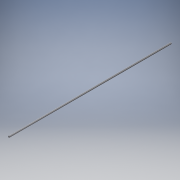
# Autodesk Inventor part: PIVOT WIRE
Saved by Autodesk Inventor 2016 (Build 200138000, 138)
## iProperties
Created: 2015-09-17
Part Number: PIVOT WIRE
Material: Steel, Mild
Document SubType Name: Modeling
Designer: testing
Density: 7.86 g/cm^3
Appearance: Metal-Steel
Author: testing
Autodesk Inventor part; units mm, degrees
ref_plane "YZ Plane" through (0, 0, 0) normal (1, 0, 0) x (0, 1, 0)
ref_plane "XZ Plane" through (0, 0, 0) normal (0, 1, 0) x (-1, 0, 0)
ref_plane "XY Plane" through (0, 0, 0) normal (0, 0, 1) x (1, 0, 0)
sketch "Sketch2" plane through (0, 0, 0) normal (0, 1, 0) x (-1, 0, 0)
  circle A0 centre (0, 0) radius 1.5
  dimension "d5" = 3
  constraints: 1 centre point, 1 coincident
  measures "d5" diameter of A0
extrude "Extrusion1" add sketch "Sketch2" along normal blind 304.8
chamfer "Chamfer1" distance 0.2 angle 45 2 edges at (1.5, 0, 0) (1.5, 304.8, 0)
body "Solid1"
